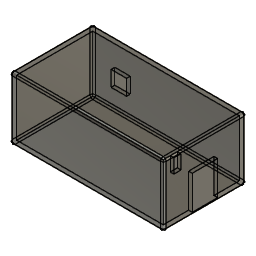
SesnsorsCase (Autodesk Fusion 360 design; units mm, degrees)
part number: 2026-04-09-15-29-07-697
Autodesk Fusion 360 part; units mm, degrees
sketch "Boceto1" plane through (0, 0, 0) normal (0, 0, 1) x (1, 0, 0)
  line L0 (0, 0) -> (104, 0)
  line L1 (104, 0) -> (104, 54)
  line L2 (104, 54) -> (0, 54)
  line L3 (0, 54) -> (0, 0)
  dimension "d1" = 104
  dimension "d2" = 54
  constraint horizontal L0
  constraint vertical L1
  constraint horizontal L2
  constraint vertical L3
  constraint coincident L0.start L3.end
  measures "d1" distance of L0.start L0.end
  measures "d2" distance of L0.start L2.end
extrude "Extruir1" add sketch "Boceto1" along normal blind 40
shell "Vaciado1" thickness 2.6 outward yes removed faces 0 bodies 1
fillet "Empalme1" radius 2 12 edges at (106.6, -2.6, 20) (106.6, 27, 42.6) (52, -2.6, 42.6) (106.6, 56.6, 20) (106.6, 27, -2.6) (52, -2.6, -2.6) (52, 56.6, 42.6) (-2.6, 27, 42.6) (-2.6, -2.6, 20) (52, 56.6, -2.6) (-2.6, 56.6, 20) (-2.6, 27, -2.6)
sketch "Boceto2" plane through (104, 0, 0) normal (-1, 0, 0) x (0, -1, 0)
  line L0 (-54, 0) -> (0, 0)
  line L1 (0, 0) -> (0, 40)
  line L2 (0, 40) -> (-54, 40)
  line L3 (-54, 40) -> (-54, 0)
  line L4 (-36, 0) -> (-36, 24)
  line L5 (-36, 24) -> (-18, 24)
  line L6 (-18, 24) -> (-18, 0)
  line L7 (-5, 40) -> (-5, 30)
  line L8 (-5, 30) -> (-10, 30)
  line L9 (-10, 30) -> (-10, 40)
  line L10 (-36, 0) -> (-18, 0)
  line L11 (-10, 40) -> (-5, 40)
  dimension "d8" = 24
  dimension "d9" = 18
  dimension "d10" = 18
  dimension "d11" = 10
  dimension "d12" = 5
  dimension "d13" = 5
  constraint coincident L0 L4.start
  constraint perpendicular L0 L4
  constraint perpendicular L4 L5
  constraint coincident L0 L6.end
  constraint perpendicular L0 L6
  constraint coincident L2 L7.start
  constraint perpendicular L2 L7
  constraint perpendicular L7 L8
  constraint coincident L2 L9.end
  constraint perpendicular L2 L9
  measures "d8" distance of L4.start L4.end
  measures "d9" distance of L4.end L5.end
  measures "d10" distance of L3 L4
  measures "d11" distance of L7.start L7.end
  measures "d12" distance of L7.end L8.end
  measures "d13" distance of L1 L7
extrude "Extruir2" cut sketch "Boceto2" against normal blind 5 contours L0 L4 L5 L6 L10 | L2 L7 L8 L9 L11
sketch "Boceto3" plane through (0, 54, 0) normal (0, -1, 0) x (1, 0, 0)
  line L0 (0, 0) -> (104, 0)
  line L1 (104, 0) -> (104, 40)
  line L2 (104, 40) -> (0, 40)
  line L3 (0, 40) -> (0, 0)
  line L4 (13, 23) -> (24, 23)
  line L5 (24, 23) -> (24, 12)
  line L6 (24, 12) -> (13, 12)
  line L7 (13, 12) -> (13, 23)
  dimension "d16" = 11
  dimension "d17" = 11
  dimension "d18" = 13
  dimension "d19" = 12
  constraint horizontal L4
  constraint vertical L5
  constraint horizontal L6
  constraint vertical L7
  measures "d16" distance of L4.start L4.end
  measures "d17" distance of L4.start L6.end
  measures "d18" distance of L3 L7
  measures "d19" distance of L0 L6
extrude "Extruir3" cut sketch "Boceto3" against normal blind 15 contours L4 L5 L6 L7
named bodies: "Case"
